Fin 3 upper part_v4 (Autodesk Fusion 360 design; units mm, degrees)
Autodesk Fusion 360 part; units mm, degrees
note: some values were not read from the file. Chosen so that the rebuilt part matches the saved one: which face or edge a step refers to.
sketch "Bottom Sketch" plane through (0, 0, 0) normal (0, 0, 1) x (1, 0, 0)
  line L0 (0, 0) -> (-160, 0)
  line L1 (-160, 0) -> (-160, 120)
  line L2 (-160, 120) -> (0, 120)
  line L3 (0, 120) -> (0, 0)
  line L4 (-160, 0) -> (-145, 0)
  line L5 (-145, 0) -> (-145, 3.175)
  line L6 (-145, 3.175) -> (-135, 3.175)
  line L7 (-135, 3.175) -> (-135, 0)
  circle A0 centre (-144.399, 2.574) radius 1
  circle A1 centre (-135.601, 2.574) radius 1
  line L8 (-160, 15) -> (-156.825, 15)
  line L9 (-156.825, 15) -> (-156.825, 25)
  line L10 (-156.825, 25) -> (-160, 25)
  circle A2 centre (-157.426, 24.399) radius 1
  circle A3 centre (-157.426, 15.601) radius 1
  line L11 (-202, -0.5275) -> (-202, 3.175)
  line L12 (-212, 120) -> (-162, 120)
  line L13 (-162, 120) -> (-162, 0)
  line L14 (-202, 3.175) -> (-192, 3.175)
  circle A4 centre (-201.399, 2.574) radius 1
  line L15 (-192, 3.175) -> (-192, 0)
  circle A5 centre (-192.601, 2.574) radius 1
  line L16 (-212, 0) -> (-212, 120)
  line L17 (-162, 0) -> (-212, 0)
  line L18 (-37.9758, 24.6213) -> (-16.7639, 24.6213) construction
  line L19 (-16.7639, 24.6213) -> (-16.7639, 31.6213) construction
  line L20 (-16.7639, 31.6213) -> (-37.9758, 31.6213) construction
  line L21 (-37.9758, 31.6213) -> (-37.9758, 24.6213) construction
  line L22 (-124.2042, 23.5425) -> (-110.7989, 23.5425) construction
  line L23 (-110.7989, 23.5425) -> (-110.7989, 30.5425) construction
  line L24 (-110.7989, 30.5425) -> (-124.2042, 30.5425) construction
  line L25 (-124.2042, 30.5425) -> (-124.2042, 23.5425) construction
  line L26 (-165.175, 0) -> (-165.175, 15)
  line L27 (-165.175, 15) -> (-162, 15)
  line L28 (-162, 120) -> (-75.7458, 120)
  line L29 (-162, 120) -> (-165.175, 120)
  line L30 (-165.175, 120) -> (-165.175, 105)
  line L31 (-165.175, 105) -> (-162, 105)
  line L32 (-162, 105) -> (-162, 120)
  line L33 (-162, 25) -> (-165.175, 25)
  line L34 (-165.175, 25) -> (-165.175, 35)
  line L35 (-165.175, 35) -> (-162, 35)
  line L36 (-162, 35) -> (-162, 25)
  circle A6 centre (-164.574, 25.601) radius 1
  circle A7 centre (-164.574, 34.399) radius 1
  circle A8 centre (-164.574, 14.399) radius 1
  line L37 (0, 162) -> (0, 172)
  line L38 (0, 172) -> (0, 122)
  line L39 (-160, 122) -> (-160, 172)
  line L40 (-145, 125.175) -> (-145, 122)
  line L41 (0, 152) -> (0, 142)
  line L42 (-135, 122) -> (-135, 125.175)
  line L43 (-160, 122) -> (-135, 122)
  line L44 (-3.175, 132) -> (0, 132)
  line L45 (-3.175, 162) -> (0, 162)
  line L46 (0, 122) -> (-160, 122)
  line L47 (-3.175, 142) -> (-3.175, 152)
  line L48 (-3.175, 172) -> (-3.175, 162)
  line L49 (0, 172) -> (-19.1943, 172)
  circle A9 centre (-134.399, 124.574) radius 1
  line L50 (-160, 125.175) -> (-145, 125.175)
  circle A10 centre (-2.574, 142.601) radius 1
  line L51 (-160, 172) -> (0, 172)
  line L52 (0, 172) -> (-3.175, 172)
  line L53 (-135, 125.175) -> (-125, 125.175)
  circle A11 centre (-145.601, 124.574) radius 1
  line L54 (-3.175, 122) -> (-3.175, 132)
  line L55 (-3.175, 152) -> (0, 152)
  line L56 (-35.0379, 97.9065) -> (-21.6326, 97.9065) construction
  line L57 (-21.6326, 97.9065) -> (-21.6326, 104.9065) construction
  line L58 (-21.6326, 104.9065) -> (-35.0379, 104.9065) construction
  line L59 (-35.0379, 104.9065) -> (-35.0379, 97.9065) construction
  line L60 (-125, 125.175) -> (-125, 122)
  circle A12 centre (-125.601, 124.574) radius 1
  line L61 (0, 142) -> (-3.175, 142)
  circle A13 centre (-2.574, 151.399) radius 1
  circle A14 centre (-2.574, 131.399) radius 1
  line L62 (0, 125.175) -> (-15, 125.175)
  line L63 (-15, 125.175) -> (-15, 122)
  circle A15 centre (-164.574, 105.601) radius 1
  circle A16 centre (-14.399, 124.574) radius 1
  circle A17 centre (-2.574, 162.601) radius 1
  circle A18 centre (-80, 142) radius 3.5
  line L64 (-117, 157) -> (-140, 157)
  line L65 (-140, 157) -> (-140, 149)
  line L66 (-140, 149) -> (-117, 149)
  line L67 (-117, 149) -> (-117, 157)
  line L68 (-117, 157) -> (-140, 149) construction
  line L69 (-140, 157) -> (-117, 149) construction
  line L70 (-35, 139) -> (-20, 139)
  line L71 (-20, 139) -> (-20, 132)
  line L72 (-20, 132) -> (-35, 132)
  line L73 (-35, 132) -> (-35, 139)
  point P0 (-128.5, 153)
  dimension "d8" = 120
  dimension "d12" = 10
  dimension "d13" = 3.175
  dimension "d14" = 3.175
  dimension "d34" = 2
  dimension "d36" = 0.601
  dimension "d37" = 0.601
  dimension "d38" = 0.601
  dimension "d48" = 2
  dimension "d49" = 0.601
  dimension "d50" = 15
  dimension "d51" = 3.175
  dimension "d52" = 0.601
  dimension "d54" = 0.601
  dimension "d55" = 10
  dimension "d80" = 120
  dimension "d82" = 10
  dimension "d85" = 50
  dimension "d86" = 2
  dimension "d87" = 0.601
  dimension "d88" = 0.601
  dimension "d89" = 0.601
  dimension "d98" = 2
  dimension "d99" = 15
  dimension "d100" = 3.175
  dimension "d104" = 3.175
  dimension "d105" = 10
  dimension "d106" = 25
  dimension "d113" = 2
  dimension "d114" = 0.601
  dimension "d115" = 0.601
  dimension "d116" = 2
  dimension "d117" = 0.601
  dimension "d119" = 0.601
  dimension "d122" = 10
  dimension "d140" = 50
  dimension "d141" = 10
  dimension "d142" = 3.175
  dimension "d143" = 3.175
  dimension "d144" = 160
  dimension "d145" = 2
  dimension "d146" = 0.601
  dimension "d147" = 0.601
  dimension "d148" = 0.601
  dimension "d149" = 10
  dimension "d150" = 3.175
  dimension "d151" = 3.175
  dimension "d152" = 10
  dimension "d154" = 2
  dimension "d155" = 0.601
  dimension "d156" = 0.601
  dimension "d157" = 2
  dimension "d158" = 0.601
  dimension "d159" = 0.601
  dimension "d160" = 3.175
  dimension "d163" = 2
  dimension "d164" = 0.601
  dimension "d165" = 2
  dimension "d171" = 10
  dimension "d177" = 160
  dimension "d182" = 0.601
  dimension "d183" = 3.175
  dimension "d184" = 2
  dimension "d185" = 2
  dimension "d186" = 0.601
  dimension "d187" = 0.601
  dimension "d189" = 15
  dimension "d191" = 15
  dimension "d192" = 10
  dimension "d193" = 15
  dimension "d247" = 7
  dimension "d248" = 23
  dimension "d249" = 8
  dimension "d250" = 30
  dimension "d251" = 80
  dimension "d253" = 20
  dimension "d254" = 15
  dimension "d255" = 15
  dimension "d256" = 7
  dimension "d257" = 10
  dimension "d258" = 20
  constraint horizontal L0
  constraint vertical L1
  constraint horizontal L2
  constraint vertical L3
  constraint coincident L0.start L3.end
  constraint horizontal L4
  constraint perpendicular L4 L5
  constraint perpendicular L5 L6
  constraint perpendicular L6 L7
  constraint equal A0 A1
  constraint horizontal A0.centre A1.centre
  constraint coincident L1 L8.start
  constraint perpendicular L1 L8
  constraint perpendicular L8 L9
  constraint coincident L1 L10.end
  constraint perpendicular L1 L10
  constraint equal A2 A3
  constraint vertical A2.centre A3.centre
  constraint horizontal L17
  constraint vertical L16
  constraint horizontal L12
  constraint vertical L13
  constraint perpendicular L11 L14
  constraint perpendicular L14 L15
  constraint equal A4 A5
  constraint horizontal A4.centre A5.centre
  constraint perpendicular L18 L19
  constraint parallel L18 L20
  constraint parallel L19 L21
  constraint perpendicular L22 L23
  constraint parallel L22 L24
  constraint parallel L23 L25
  constraint coincident L17 L26.start
  constraint perpendicular L17 L26
  constraint coincident L13 L27.end
  constraint perpendicular L13 L27
  constraint coincident L12 L28.end
  constraint perpendicular L13 L28
  constraint horizontal L29
  constraint vertical L30
  constraint horizontal L31
  constraint vertical L32
  constraint equal L27 L31
  constraint equal L26 L30
  constraint horizontal L33
  constraint vertical L34
  constraint horizontal L35
  constraint vertical L36
  constraint coincident L13 L33.start
  constraint equal A6 A7
  constraint vertical A6.centre A7.centre
  constraint vertical A7.centre A8.centre
  constraint collinear L0 L17
  constraint horizontal L46
  constraint vertical L39
  constraint horizontal L51
  constraint vertical L38
  constraint horizontal L43
  constraint perpendicular L42 L43
  constraint perpendicular L42 L53
  constraint perpendicular L53 L60
  constraint equal A9 A12
  constraint horizontal A12.centre A9.centre
  constraint perpendicular L56 L57
  constraint parallel L56 L58
  constraint parallel L57 L59
  constraint coincident L54.start L46
  constraint perpendicular L46 L54
  constraint coincident L44.end L38
  constraint perpendicular L38 L44
  constraint coincident L49.end L51
  constraint perpendicular L38 L49
  constraint horizontal L52
  constraint vertical L48
  constraint horizontal L45
  constraint vertical L37
  constraint equal L44 L45
  constraint equal L48 L54
  constraint horizontal L61
  constraint vertical L47
  constraint horizontal L55
  constraint vertical L41
  constraint coincident L41.end L38
  constraint equal A10 A13
  constraint vertical A13.centre A10.centre
  constraint vertical A14.centre A13.centre
  constraint coincident L50.start L39
  constraint perpendicular L39 L50
  constraint coincident L40.end L43
  constraint perpendicular L40 L43
  constraint horizontal A9.centre A11.centre
  constraint collinear L1 L39
  constraint coincident L38 L62.start
  constraint coincident L46 L63.end
  constraint perpendicular L46 L63
  constraint collinear L50 L62
  constraint vertical A7.centre A15.centre
  constraint equal A7 A15
  constraint horizontal A12.centre A16.centre
  constraint vertical A14.centre A17.centre
  constraint horizontal L64
  constraint perpendicular L64 L65
  constraint parallel L64 L66
  constraint parallel L65 L67
  constraint coincident L68 P0
  constraint coincident L69 P0
  constraint horizontal L70
  constraint vertical L71
  constraint horizontal L72
  constraint vertical L73
  measures "d8" distance of L0.start L2.end
  measures "d12" distance of L5.end L6.end
  measures "d13" distance of L4.end L5.end
  measures "d14" distance of L6.end L7.end
  measures "d34" diameter of A0
  measures "d36" distance of L5 A0.centre
  measures "d37" distance of L6 A0.centre
  measures "d38" horizontal distance of L7.end A1.centre
  measures "d48" diameter of A2
  measures "d49" distance of L8 A3.centre
  measures "d50" distance of L4 L8
  measures "d51" distance of L9.end L10.end
  measures "d52" distance of L10 A2.centre
  measures "d54" distance of L9 A3.centre
  measures "d55" distance of L8 L10
  measures "d80" distance of L13.end L12.end
  measures "d82" distance of L11.end L14.end
  measures "d85" distance of L12.start L12.end
  measures "d86" diameter of A4
  measures "d87" distance of A4.centre L11
  measures "d88" distance of A4.centre L14
  measures "d89" horizontal distance of A5.centre L15.end
  measures "d98" distance of L0.end L13.end
  measures "d99" distance of L17 L27
  measures "d100" distance of L13 L26
  measures "d104" distance of L34.end L35.end
  measures "d105" distance of L33.end L34.end
  measures "d106" distance of L17 L33
  measures "d113" diameter of A6
  measures "d114" distance of L34 A6.centre
  measures "d115" distance of L33 A6.centre
  measures "d116" diameter of A8
  measures "d117" distance of L35 A7.centre
  measures "d119" distance of L27 A8.centre
  measures "d122" distance of L11 L16
  measures "d140" distance of L37.end L38.end
  measures "d141" distance of L53.end L42.end
  measures "d142" distance of L42.start L42.end
  measures "d143" distance of L53.end L60.end
  measures "d144" distance of L37.end L39.end
  measures "d145" diameter of A9
  measures "d146" distance of A9.centre L42
  measures "d147" distance of A9.centre L53
  measures "d148" horizontal distance of A12.centre L60.end
  measures "d149" distance of L44 L46
  measures "d150" distance of L38 L54
  measures "d151" distance of L47.end L41.start
  measures "d152" distance of L47.start L47.end
  measures "d154" diameter of A10
  measures "d155" distance of A10.centre L47
  measures "d156" distance of A10.centre L61
  measures "d157" diameter of A14
  measures "d158" distance of A13.centre L55
  measures "d159" distance of A14.centre L44
  measures "d160" distance of L43 L50
  measures "d163" diameter of A11
  measures "d164" distance of A11.centre L40
  measures "d165" distance of L2 L46
  measures "d171" distance of L44 L61
  measures "d177" distance of L1 L3
  measures "d182" vertical distance of L30.end A15.centre
  measures "d183" distance of L14 L17
  measures "d184" diameter of A17
  measures "d185" diameter of A16
  measures "d186" distance of L45 A17.centre
  measures "d187" distance of L63 A16.centre
  measures "d189" distance of L1 L5
  measures "d191" distance of L39 L40
  measures "d192" distance of L40 L42
  measures "d193" distance of L38 L63
  measures "d247" diameter of A18
  measures "d248" distance of L65.end L66.end
  measures "d249" distance of L64.end L65.end
  measures "d250" distance of L51 A18.centre
  measures "d251" distance of L39 A18.centre
  measures "d253" distance of L39 L65
  measures "d254" distance of L51 L64
  measures "d255" distance of L70.start L70.end
  measures "d256" distance of L70.start L72.end
  measures "d257" distance of L46 L72
  measures "d258" distance of L38 L71
extrude "extrude bottom" add sketch "Bottom Sketch" along normal blind 3.175 contours L0 L1 L2 L3 L4 L5 L6 L7 A0 A1 L8 L9 L10 A2 A3 L28 makes body 1
pattern_linear "bottom length repeat fingers" count 7 spacing 20 along (1, 0, 0) of 6 faces at (-144.1695, 3.5473, 2.1167) (-145, 0.5916, 1.0583) (-141.1999, 3.175, 1.0583) (-135, 1.1832, 1.0583) (-134.8398, 1.9255, 2.1167) (-135.7432, 3.5638, 2.1167) on bodies 1
pattern_linear "bottom depth repeat fingers" count 5 spacing 20 along (0, 1, 0) of 5 faces at (-159.4084, 15, 1.0583) (-157.5086, 14.6045, 1.0583) (-156.825, 18.8001, 1.0583) (-157.558, 25.3902, 2.1167) (-158.8168, 25, 1.0583) on bodies 1
extrude "extrude side" add sketch "Bottom Sketch" along normal blind 3.175 separate body contours L11 L12 L13 L14 A4 L15 A5 L16 L17 L26 L27 L30 L31 L33 L34 L35 A6 A7 A8 A15 makes body 2
pattern_linear "side height repeat fingers" count 2 spacing 20 along (1, 0, 0) of 6 faces at (-202, 0.5916, 1.0583) (-200.7717, 3.3528, 2.1167) (-198.1999, 3.175, 1.0583) (-191.7609, 2.0316, 2.1167) (-192.6946, 3.5696, 2.1167) (-192, 1.1832, 1.0583) on bodies 2
pattern_linear "side depth repeat fingers" count 5 spacing 20 along (0, 1, 0) of 5 faces at (-163.1832, 35, 1.0583) (-164.1571, 35.308, 2.1167) (-165.175, 28.8001, 1.0583) (-164.442, 24.6098, 2.1167) (-163.1832, 25, 2.1167) on bodies 2
extrude "Extrude Face" add sketch "Bottom Sketch" along normal blind 3.175 separate body contours L38 L39 L40 L42 L43 L44 L45 L46 L47 L48 L49 A9 L50 A10 L51 L53 A11 L54 L55 L60 A12 L61 A13 A14 L62 L63 A16 A17 | A18 | L64 L65 L66 L67 | L70 L71 L72 L73 makes body 3
pattern_linear "front length repeat finger holes" count 6 spacing 20 along (1, 0, 0) of 6 faces at (-135, 122.5916, 1.0583) (-134.0277, 125.5025, 2.1167) (-131.1999, 125.175, 1.0583) (-124.6166, 124.3985, 2.1167) (-125.0433, 125.404, 2.1167) (-125, 123.1832, 1.0583) on bodies 3
pattern_linear "front height repeat finger holes" count 2 spacing 20 along (0, 1, 0) of 5 faces at (-0.5916, 142, 1.0583) (-3.525, 142.292, 2.1167) (-3.175, 145.8001, 1.0583) (-3.5705, 151.3164, 2.1167) (-1.1832, 152, 1.0583) on bodies 3
ref_plane "WorkPlane5" through (-67.5, 60, 1.5875) normal (0, -1, 0) x (1, 0, 0)
mirror "Mirror Bottom on X" about plane through (-67.5, 60, 1.5875) normal (0, -1, 0) of bodies 1 makes body 4
combine "Combine5" operation intersect target body 1 tool bodies 4
ref_plane "WorkPlane6" through (-80, 60, 1.5875) normal (1, 0, 0) x (0, 1, 0)
mirror "Mirror Bottom on Y" about plane through (-80, 60, 1.5875) normal (1, 0, 0) of bodies 1 makes body 5
combine "Combine6" operation intersect target body 1 tool bodies 5
ref_plane "WorkPlane7" through (-178.5875, 60, 1.5875) normal (0, -1, 0) x (1, 0, 0)
mirror "Mirror SIde on X" about plane through (-178.5875, 60, 1.5875) normal (0, -1, 0) of bodies 2 makes body 6
combine "Combine7" operation intersect target body 6 tool bodies 2
ref_plane "WorkPlane8" through (-187, 60, 1.5875) normal (-1, 0, 0) x (0, 1, 0)
mirror "Mirror10" about plane through (-187, 60, 1.5875) normal (-1, 0, 0) of bodies 6 makes body 7
combine "Combine8" operation intersect target body 6 tool bodies 7
ref_plane "WorkPlane9" through (-70, 147, 1.5875) normal (0, -1, 0) x (1, 0, 0)
mirror "Mirror1 Face on X" about plane through (-70, 147, 1.5875) normal (0, -1, 0) of bodies 3 makes body 8
combine "Combine9" operation intersect target body 3 tool bodies 8
ref_plane "WorkPlane11" through (-80, 147, 1.5875) normal (-1, 0, 0) x (0, -1, 0)
mirror "Mirror12" about plane through (-80, 147, 1.5875) normal (-1, 0, 0) of bodies 3 makes body 9
combine "Combine10" operation intersect target body 3 tool bodies 9
sketch "Stock" plane through (0, 0, 0) normal (0, 0, 1) x (1, 0, 0)
  line L0 (0, 0) -> (-609.6, 0)
  line L1 (-609.6, 0) -> (-609.6, 304.8)
  line L2 (-609.6, 304.8) -> (0, 304.8)
  line L3 (0, 304.8) -> (0, 0)
  dimension "d206" = 609.6
  dimension "d207" = 304.8
  constraint horizontal L0
  constraint vertical L1
  constraint horizontal L2
  constraint vertical L3
  constraint coincident L0.start L3.end
  measures "d206" distance of L0.start L0.end
  measures "d207" distance of L0.end L1.end
copy_body "CopyPasteBodies4" bodies 1 makes body 10
move_body "Move6" bodies 10 to x (1, 0, 0) y (0, 1, 0) z (0, 0, 1) at (0, 174, 0)
copy_body "CopyPasteBodies5" bodies 6 makes body 11
move_body "Move7" bodies 11 to x (1, 0, 0) y (0, 1, 0) z (0, 0, 1) at (0, 122, 0)
copy_body "CopyPasteBodies6" bodies 3 makes body 12
move_body "Move20" bodies 12 to x (0, 1, 0) y (-1, 0, 0) z (0, 0, 1) at (0, 0, 0)
move_body "Move21" bodies 12 to x (1, 0, 0) y (0, 1, 0) z (0, 0, 1) at (-93, 300, 0)
move_body "Move22" bodies 3 10 1 6 11 to x (1, 0, 0) y (0, 1, 0) z (0, 0, 1) at (-350, 0, 0)
move_body "Move23" bodies 11 to x (1, 0, 0) y (0, 1, 0) z (0, 0, 1) at (500, 50, 0)
move_body "Align1" bodies 12 to x (1, 0, 0) y (0, 1, 0) z (0, 0, 1) at (218.175, -143.175, 0)
move_body "Move24" bodies 12 to x (1, 0, 0) y (0, 1, 0) z (0, 0, 1) at (-6.35, 6.35, 0)
move_body "Align2" bodies 11 to x (1, 0, 0) y (0, 1, 0) z (0, 0, 1) at (8.825, -12, 0)
move_body "Move25" bodies 11 to x (1, 0, 0) y (0, 1, 0) z (0, 0, 1) at (0, 8, 0)
copy_body "CopyPasteBodies7" bodies 12 11 makes body 13 makes body 14
move_body "Move26" bodies 13 14 to x (1, 0, 0) y (0, 1, 0) z (0, 0, 1) at (-52, 0, 0)
delete_body "RemoveBody1" bodies 1
delete_body "RemoveBody2" bodies 10
delete_body "RemoveBody3" bodies 3
delete_body "RemoveBody4" bodies 6
move_face "MoveFace5" by (0, -10, 0) 2 faces at (-78.4054, 269.7905, 3.175) (-78.8084, 144.9366, 3.175) on bodies 13 14
move_body "Move27" bodies 14 13 to x (1, 0, 0) y (0, 1, 0) z (0, 0, 1) at (-20, 0, 0)
delete_body "RemoveBody5" bodies 13
delete_body "RemoveBody6" bodies 14
sketch "Sketch8" plane through (0, 0, 0) normal (0, 0, 1) x (1, 0, 0)
  circle A0 centre (-35.175, 93.175) radius 3.5
  line L0 (-43.175, 3.175) -> (-33.175, 3.175)
  line L1 (-41.675, 46.175) -> (-31.175, 46.175)
  line L2 (-31.175, 46.175) -> (-31.175, 23.175)
  line L3 (-31.175, 23.175) -> (-41.675, 23.175)
  line L4 (-41.675, 23.175) -> (-41.675, 46.175)
  line L5 (-53.175, 28.175) -> (-53.175, 18.175)
  line L6 (-23.175, 148.175) -> (-15.175, 148.175)
  line L7 (-15.175, 148.175) -> (-15.175, 133.175)
  line L8 (-15.175, 133.175) -> (-23.175, 133.175)
  line L9 (-23.175, 133.175) -> (-23.175, 148.175)
  line L10 (-13.175, 163.175) -> (-23.175, 163.175)
  line L11 (-3.175, 138.175) -> (-3.175, 148.175)
  point P0 (-53.175, 78.175)
  dimension "d265" = 90
  dimension "d266" = 7
  dimension "d267" = 18
  dimension "d268" = 10.5
  dimension "d269" = 23
  dimension "d270" = 20
  dimension "d271" = 22
  dimension "d272" = 15
  dimension "d273" = 8
  dimension "d274" = 15
  dimension "d275" = 12
  constraint horizontal L1
  constraint vertical L2
  constraint horizontal L3
  constraint vertical L4
  constraint horizontal L6
  constraint vertical L7
  constraint horizontal L8
  constraint vertical L9
  measures "d265" distance of A0.centre L0
  measures "d266" diameter of A0
  measures "d267" horizontal distance of A0.centre P0
  measures "d268" distance of L1.start L1.end
  measures "d269" distance of L1.start L3.end
  measures "d270" distance of L0.start L3
  measures "d271" distance of L2 L5
  measures "d272" distance of L6.start L8.end
  measures "d273" distance of L7.end L8.end
  measures "d274" distance of L6 L10
  measures "d275" distance of L7 L11
extrude "Extrude7" cut sketch "Sketch8" along normal blind 3.175 contours L1 L2 L3 L4 | L6 L7 L8 L9 bodies 12
extrude "Extrude6" cut sketch "Sketch8" along normal blind 3.175 contours A0 bodies 12
equation "fingerWidth = 10 mm"
equation "length = 160 mm"
equation "thickness = 3.175 mm"
equation "height = 50 mm"
equation "d8 = depth"
equation "d12 = fingerWidth"
equation "d13 = thickness"
equation "d14 = thickness"
equation "d15 = thickness"
equation "d21 = lengthCutsBottom"
equation "d23 = -2 * fingerWidth"
equation "toolDiameter = 2 mm"
equation "d34 = toolDiameter"
equation "d36 = cornerToCenterForBone"
equation "d37 = cornerToCenterForBone"
equation "d38 = cornerToCenterForBone"
equation "cornerToCenterForBone = toolDiameter / 2 / sqrt(2) * reduceBone"
equation "tempLengthPiecesBottom = ceil(( ( floor(( length - 2 * thickness ) / fingerWidth) - 2 ) - ( ( floor(( length - 2 * thickness ) / fingerWidth) - 2 ) % 2 - 1 ) ))"
equation "lengthCutsBottom = ceil(tempLengthPiecesBottom / 2)"
equation "lengthShoulder = ( length - fingerWidth * tempLengthPiecesBottom ) / 2"
equation "depth = 120 mm"
equation "tempDepthPiecesBottom = ceil(( ( floor(( depth - 2 * thickness ) / fingerWidth) - 2 ) - ( ( floor(( depth - 2 * thickness ) / fingerWidth) - 2 ) % 2 - 1 ) ))"
equation "depthCutsSideBottom = ceil(tempDepthPiecesBottom / 2)"
equation "depthShoulder = ( depth - fingerWidth * tempDepthPiecesBottom ) / 2"
equation "d48 = toolDiameter"
equation "d49 = cornerToCenterForBone"
equation "d50 = depthShoulder"
equation "d51 = thickness"
equation "d52 = cornerToCenterForBone"
equation "d54 = cornerToCenterForBone"
equation "d55 = fingerWidth"
equation "d56 = depthCutsSideBottom"
equation "d58 = 2 * fingerWidth"
equation "d80 = depth"
equation "d82 = fingerWidth"
equation "d85 = height"
equation "d86 = toolDiameter"
equation "d87 = cornerToCenterForBone"
equation "d88 = cornerToCenterForBone"
equation "d89 = cornerToCenterForBone"
equation "d98 = toolDiameter"
equation "d99 = depthShoulder"
equation "d100 = thickness"
equation "tempHeightPiecesSide = ceil(( ( floor(( height - 2 * thickness ) / fingerWidth) - 2 ) - ( ( floor(( height - 2 * thickness ) / fingerWidth) - 2 ) % 2 - 1 ) ))"
equation "heightCutsSide = ceil(tempHeightPiecesSide / 2)"
equation "heightSholder = ( height - fingerWidth * tempHeightPiecesSide ) / 2"
equation "d104 = thickness"
equation "d105 = fingerWidth"
equation "d106 = depthShoulder + fingerWidth"
equation "d113 = toolDiameter"
equation "d114 = cornerToCenterForBone"
equation "d115 = cornerToCenterForBone"
equation "d116 = toolDiameter"
equation "d117 = cornerToCenterForBone"
equation "d119 = cornerToCenterForBone"
equation "d122 = heightSholder"
equation "d126 = thickness"
equation "d128 = heightCutsSide"
equation "d130 = -2 * fingerWidth"
equation "d132 = depthCutsSideBottom"
equation "d134 = -2 * fingerWidth"
equation "d140 = height"
equation "d141 = fingerWidth"
equation "d142 = thickness"
equation "d143 = thickness"
equation "d144 = length"
equation "d145 = toolDiameter"
equation "d146 = cornerToCenterForBone"
equation "d147 = cornerToCenterForBone"
equation "d148 = cornerToCenterForBone"
equation "d149 = heightSholder"
equation "d150 = thickness"
equation "d151 = thickness"
equation "d152 = fingerWidth"
equation "d154 = toolDiameter"
equation "d155 = cornerToCenterForBone"
equation "d156 = cornerToCenterForBone"
equation "d157 = toolDiameter"
equation "d158 = cornerToCenterForBone"
equation "d159 = cornerToCenterForBone"
equation "d160 = thickness"
equation "d163 = toolDiameter"
equation "d164 = cornerToCenterForBone"
equation "d165 = toolDiameter"
equation "d169 = thickness"
equation "d171 = fingerWidth"
equation "d172 = lengthCutsBottom - 1"
equation "d174 = -2 * fingerWidth"
equation "d177 = length"
equation "d178 = heightCutsSide"
equation "d180 = -2 * fingerWidth"
equation "d182 = cornerToCenterForBone"
equation "d183 = thickness"
equation "d184 = toolDiameter"
equation "d185 = toolDiameter"
equation "d186 = cornerToCenterForBone"
equation "d187 = cornerToCenterForBone"
equation "d189 = lengthShoulder"
equation "d191 = lengthShoulder"
equation "d192 = fingerWidth"
equation "d193 = lengthShoulder"
equation "d215 = depth + height + 2 * toolDiameter"
equation "d218 = depth + toolDiameter"
equation "d237 = -thickness * 2"
equation "d238 = thickness * 2"
equation "d241 = toolDiameter * 4"
equation "d243 = -height - toolDiameter"
equation "reduceBone = 0.85"
equation "d250 = height / 2 + 5 mm"
equation "d251 = length / 2"
equation "d265 = length / 2 + 10 mm"
equation "d267 = height / 2 - 7 mm"
equation "d276 = thickness"
named bodies: "Side", "Front", "Bottom", "Bottom (1)", "Side (1) (1)", "Face (1)", "Side (1)", "Face", "Front (1)", "Front (1) (1)"
